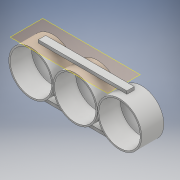
# Autodesk Inventor part: receptacle
Saved by Autodesk Inventor 2018 (Build 220112000, 112)
## iProperties
Created: 2018-04-09
Part Number: receptacle
Material: Générique
Document SubType Name: Modeling
Designer: Dimitri
Density: 1 g/cm^3
Appearance: Par défaut
Author: Dimitri
Autodesk Inventor part; units mm, degrees
ref_plane "YZ Plane" through (0, 0, 0) normal (1, 0, 0) x (0, 1, 0)
ref_plane "XZ Plane" through (0, 0, 0) normal (0, 1, 0) x (-1, 0, 0)
sketch "Esquisse2" plane through (0, 0, 0) normal (0, 1, 0) x (-1, 0, 0)
  circle A0 centre (0, 0) radius 15
  dimension "d4" = 30
  constraints: 1 centre point, 1 coincident
  measures "d4" diameter of A0
extrude "Extrusion2" add sketch "Esquisse2" along normal blind 5
draft "Dépouille de face1" angle -65 pull direction (0, -1, 0) faces at (-14.8058, 3.3333, -2.4062) fixed edges at (15, 0, 0)
sketch "Esquisse3" plane through (0, 0, 0) normal (0, -1, 0) x (1, 0, 0)
  circle A0 centre (0, 0) radius 15
  dimension "d17" = 30
  constraints: 1 centre point, 1 coincident
  measures "d17" diameter of A0
extrude "Extrusion3" add sketch "Esquisse3" along normal blind 15
shell "Coque1" thickness 1 removed faces 1 at (4.7094, -15, 0)
pattern_linear "Réseau rectangulaire1" count 3 spacing 30 along (1, 0, 0) of "Extrusion2", "Dépouille de face1", "Extrusion3"
shell "Coque2" thickness 1 removed faces 2 at (25.5727, -15, 0.0695) at (55.5727, -15, 0.0695)
ref_plane "Plan de construction1" through (0, 0, 15) normal (0, 0, 1) x (1, 0, 0)
sketch "Esquisse5" plane through (0, 0, 15) normal (0, 0, 1) x (1, 0, 0)
  line L0 (-15, 0) -> (-15, -15) projected
  line L1 (-15, 0) -> (15, 0) projected
  line L2 (75, 0) -> (75, -15) projected
  line L3 (45, -15) -> (75, -15) projected
  line L4 (0, -10) -> (60, -10)
  line L5 (60, -10) -> (60, -5)
  line L6 (60, -5) -> (0, -5)
  line L7 (0, -5) -> (0, -10)
  line L8 (15, 0) -> (45, 0) projected
  point P0 (0, 0)
  dimension "d18" = 15
  dimension "d20" = 15
  dimension "d21" = 5
  dimension "d22" = 5
  constraints: 8 end point, 2 parallel, 1 horizontal, 1 perpendicular
  measures "d18" distance between parallel lines of L0 L7
  measures "d20" distance between parallel lines of L2 L5
  measures "d21" distance between parallel lines of L8 L6
  measures "d22" distance between parallel lines of L3 L4
extrude "Extrusion4" add sketch "Esquisse5" along normal blind 2
mirror "Symétrie1" about plane through (0, 0, 0) normal (0, 0, 1) of "Extrusion4"
